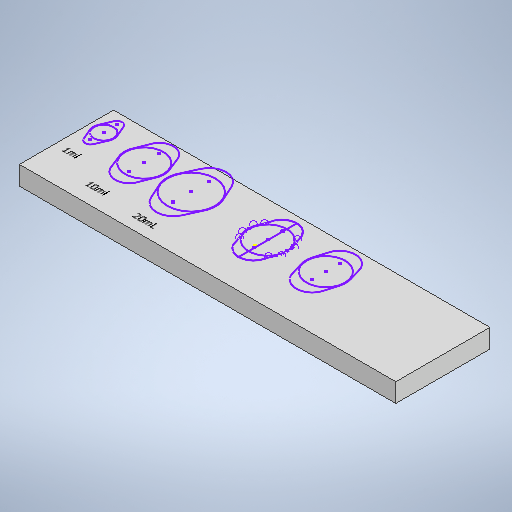
# Autodesk Inventor part: LuerLock verschiedene Größen
Saved by Autodesk Inventor 2025 (Build 290162000, 162)
## iProperties
Created: 2024-06-11
Part Number: LuerLock verschiedene Größen
Material: Generisch
Document SubType Name: Modeling
Designer: noahm
Density: 1 g/cm^3
Appearance: Vorgabe
Author: noahm
Autodesk Inventor part; units mm, degrees
ref_plane "YZ Plane" through (0, 0, 0) normal (1, 0, 0) x (0, 1, 0)
ref_plane "XZ Plane" through (0, 0, 0) normal (0, 1, 0) x (-1, 0, 0)
ref_plane "XY Plane" through (0, 0, 0) normal (0, 0, 1) x (1, 0, 0)
sketch "Skizze1" plane through (0, 0, 0) normal (0, 0, 1) x (1, 0, 0)
  line L0 (100, -25) -> (-100, -25)
  line L1 (-100, -25) -> (-100, 25)
  line L2 (-100, 25) -> (100, 25)
  line L3 (100, 25) -> (100, -25)
  line L4 (100, -25) -> (-100, 25) construction
  line L5 (-100, -25) -> (100, 25) construction
  point P0 (0, 0)
  dimension "d0" = 200
  dimension "d1" = 50
  constraints: 12 end point, 2 midpoint, 2 parallel, 1 horizontal, 1 perpendicular
  measures "d0" distance of L1.end L2.end
  measures "d1" distance of L0.end L1.end
extrude "Extrusion1" add sketch "Skizze1" along normal blind 10
sketch "Skizze2" plane through (0, 0, 10) normal (0, 0, 1) x (1, 0, 0)
  circle A0 centre (-92.2249, 11.967) radius 5.2
  arc A1 (-94.7561, 3.8919) -> (-89.6938, 3.8919) centre (-92.2249, 4.967) ccw
  line L0 (-97.4249, 10.1754) -> (-94.7561, 3.8919)
  line L1 (-89.6938, 3.8919) -> (-87.0249, 10.1754)
  line L2 (-94.7561, 20.0421) -> (-97.4249, 13.7587)
  line L3 (-89.6938, 20.0421) -> (-87.0249, 13.7587)
  arc A2 (-94.2324, 17.0876) -> (-93.9901, 16.8583) centre (-92.2249, 18.967) ccw
  arc A3 (-90.4598, 16.8583) -> (-90.2174, 17.0876) centre (-92.2249, 18.967) ccw
  arc A4 (-89.6938, 20.0421) -> (-94.7561, 20.0421) centre (-92.2249, 18.967) ccw
  arc A5 (-97.1248, 14.4652) -> (-97.1248, 9.4688) centre (-92.2249, 11.967) ccw
  arc A6 (-87.325, 9.4688) -> (-87.325, 14.4652) centre (-92.2249, 11.967) ccw
  line L4 (-95.5124, -3.9749) -> (-87.7437, -3.9749) construction
  line L5 (-87.7437, -3.9749) -> (-87.7437, -7.6309) construction
  line L6 (-87.7437, -7.6309) -> (-95.5124, -7.6309) construction
  line L7 (-95.5124, -7.6309) -> (-95.5124, -3.9749) construction
  line L8 (-73.5848, -13.5772) -> (-63.1897, -13.5772) construction
  line L9 (-63.1897, -13.5772) -> (-63.1897, -17.3069) construction
  line L10 (-63.1897, -17.3069) -> (-73.5848, -17.3069) construction
  line L11 (-73.5848, -17.3069) -> (-73.5848, -13.5772) construction
  circle A7 centre (-67.4607, 8.8016) radius 10.2
  line L12 (-74.1057, 20.2792) -> (-77.6607, 11.2936)
  line L13 (-60.8157, 20.2792) -> (-57.2607, 11.2936)
  line L14 (-60.8157, -2.676) -> (-57.2607, 6.3096)
  line L15 (-74.1057, -2.676) -> (-77.6607, 6.3096)
  arc A8 (-77.6607, 11.2936) -> (-77.6607, 6.3096) centre (-67.4607, 8.8016) ccw
  arc A9 (-74.1057, -2.676) -> (-60.8157, -2.676) centre (-67.4607, 0.8016) ccw
  arc A10 (-60.8157, 20.2792) -> (-74.1057, 20.2792) centre (-67.4607, 16.8016) ccw
  arc A11 (-57.2607, 6.3096) -> (-57.2607, 11.2936) centre (-67.4607, 8.8016) ccw
  circle A12 centre (-41.594, 7.9046) radius 12.7
  line L16 (-49.8856, 20.9046) -> (-54.0114, 11.7529)
  line L17 (-33.3883, 21.1014) -> (-29.1767, 11.7529)
  line L18 (-33.3893, -5.2943) -> (-29.1831, 4.0358)
  line L19 (-49.7998, -5.2922) -> (-54.0114, 4.0563)
  arc A13 (-54.0114, 11.7529) -> (-54.0114, 4.0563) centre (-41.594, 7.9046) ccw
  arc A14 (-29.1831, 4.0358) -> (-29.1767, 11.7529) centre (-41.594, 7.9046) ccw
  arc A15 (-49.7998, -5.2922) -> (-33.3893, -5.2943) centre (-41.594, -1.5954) ccw
  arc A16 (-33.3883, 21.1014) -> (-49.8856, 20.9046) centre (-41.594, 17.4046) ccw
  line L20 (-46.2828, -15.7278) -> (-34.5944, -15.7278) construction
  line L21 (-34.5944, -15.7278) -> (-34.5944, -19.3753) construction
  line L22 (-34.5944, -19.3753) -> (-46.2828, -19.3753) construction
  line L23 (-46.2828, -19.3753) -> (-46.2828, -15.7278) construction
  circle A17 centre (0.8113, 6.1179) radius 10.2
  arc A18 (7.4768, 17.6061) -> (-5.8132, 17.6061) centre (0.8318, 14.1284) ccw
  line L24 (-9.6887, 6.1179) -> (-9.8605, 9.0795) construction
  spline S0 degree 3 poles (-9.6887, 6.1179) (-9.8605, 9.0795) (-7.7224, 12.6783) (-7.1197, 14.6665) knots 1 1 1 1 1.859852 1.859852 1.859852 1.859852
  spline S1 degree 3 poles (-9.6887, 6.1179) (-9.8605, 3.1562) (-7.7224, -0.4426) (-7.1197, -2.4308) knots 1 1 1 1 1.859852 1.859852 1.859852 1.859852
  line L25 (-9.6887, 6.1179) -> (-9.8605, 3.1562) construction
  line L26 (0.8318, 21.6284) -> (0.8318, -9.7992)
  spline S2 degree 3 poles (11.3522, 6.1179) (11.5521, 9.5623) (8.6275, 13.8684) (8.6275, 15.5006) knots 1 1 1 1 2 2 2 2
  line L27 (11.3522, 6.1179) -> (11.5521, 9.5623) construction
  line L28 (11.5521, 9.5623) -> (8.6275, 13.8684) construction
  line L29 (8.6275, 13.8684) -> (8.6275, 15.5006) construction
  spline S3 degree 3 poles (11.3522, 6.1179) (11.5521, 2.6735) (8.6275, -1.6326) (8.6275, -3.2649) knots 1 1 1 1 2 2 2 2
  line L30 (11.3522, 6.1179) -> (11.5521, 2.6735) construction
  line L31 (11.5521, 2.6735) -> (8.6275, -1.6326) construction
  line L32 (8.6275, -1.6326) -> (8.6275, -3.2649) construction
  arc A19 (8.679, 15.0669) -> (-7.1197, 14.6665) centre (0.8113, 13.6179) ccw
  arc A20 (-7.1197, -2.4308) -> (8.679, -2.8311) centre (0.8113, -1.3821) ccw
  arc A21 (-7.1197, -2.4308) -> (8.679, -2.8311) centre (0.8113, -1.3821) ccw
  line L33 (-9.8605, 3.1562) -> (-7.7224, -0.4426) construction
  line L34 (-7.7224, -0.4426) -> (-7.1197, -2.4308) construction
  line L35 (-9.8605, 9.0795) -> (-7.7224, 12.6783) construction
  line L36 (-7.7224, 12.6783) -> (-7.1197, 14.6665) construction
  circle A22 centre (30.7605, 7.0672) radius 10.2
  line L37 (22.4266, 15.8836) -> (20.6955, 10.058)
  line L38 (39.1541, 15.7803) -> (40.7119, 10.4168)
  line L39 (39.1507, -1.6651) -> (40.8594, 4.1927)
  line L40 (22.4079, -1.6459) -> (21.0051, 3.1836)
  line L41 (30.781, 17.5672) -> (30.781, 17.2672)
  arc A23 (20.6955, 10.058) -> (21.0051, 3.1836) centre (30.7605, 7.0672) ccw
  arc A24 (40.8211, 4.0614) -> (40.7119, 10.4168) centre (30.7605, 7.0672) ccw
  arc A25 (22.4079, -1.6459) -> (39.1507, -1.6651) centre (30.781, -0.1828) ccw
  arc A26 (39.1541, 15.7803) -> (22.4266, 15.8836) centre (30.781, 14.3172) ccw
  point P0 (0, 0)
  point P1 (-67.4607, 8.8016)
  point P2 (10.8113, 6.1179)
  point P3 (-9.3887, 6.1179)
  constraints: 53 point on circle, 36 end point, 25 centre point, 8 tangent, 7 parallel, 5 point on line, 2 vertical, 1 horizontal alignment, 1 symmetric about line, 25 other
